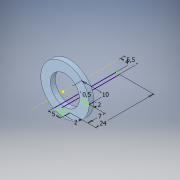
# Autodesk Inventor part: Zugentlastung
Saved by Autodesk Inventor 2018.2 (Build 222227000, 227)
## iProperties
Created: 2018-03-03
Part Number: Zugentlastung
Material: Generisch
Document SubType Name: Modeling
Designer: JochenAlt
Density: 1 g/cm^3
Appearance: Vorgabe
Author: JochenAlt
Autodesk Inventor part; units mm, degrees
ref_plane "YZ Plane" through (0, 0, 0) normal (1, 0, 0) x (0, 1, 0)
ref_plane "XZ Plane" through (0, 0, 0) normal (0, 1, 0) x (-1, 0, 0)
ref_plane "XY Plane" through (0, 0, 0) normal (0, 0, 1) x (1, 0, 0)
sketch "Skizze1" plane through (0, 0, 0) normal (0, 0, 1) x (1, 0, 0)
  line L0 (0, 23.0554) -> (0, -13.3446) construction
  line L1 (-2, 0) -> (12, 0) construction
  line L2 (4, 17.8554) -> (5.5, 17.8554)
  line L3 (5.5, 17.8554) -> (5.5, -6.1446)
  line L4 (4, 17.8554) -> (4, -8.1446)
  line L5 (4, -8.1446) -> (9, -8.1446)
  line L6 (9, -8.1446) -> (9, -6.1446)
  line L7 (9, -6.1446) -> (5.5, -6.1446)
  line L8 (6, 2.8554) -> (6, 0.8554)
  line L9 (6, 2.8554) -> (10, 2.8554)
  line L10 (10, 2.8554) -> (10, 0.8554)
  line L11 (10, 0.8554) -> (6, 0.8554)
  point P0 (0, 0)
  dimension "d9" = 4
  dimension "d10" = 5.5
  dimension "d11" = 5
  dimension "d12" = 2
  dimension "d13" = 24
  dimension "d14" = 0.5
  dimension "d15" = 2
  dimension "d16" = 10
  dimension "d21" = 7
  constraints: 20 end point, 4 perpendicular, 3 horizontal, 3 vertical
  measures "d9" distance between parallel lines of L4 L0
  measures "d10" distance between parallel lines of L0 L3
  measures "d11" distance between parallel lines of L6 L4
  measures "d12" distance between parallel lines of L5 L7
  measures "d13" distance between parallel lines of L7 L2
  measures "d14" distance between parallel lines of L3 L8
  measures "d15" distance between parallel lines of L11 L9
  measures "d16" distance between parallel lines of L10 L0
  measures "d21" distance between parallel lines of L11 L7
revolve "Umdrehung1" add sketch "Skizze1" angle 360 about axis through (0, 0, 0) along (0, -1, 0) contours L2 L3 L7 L6 L5 L4
revolve "Umdrehung2" add sketch "Skizze1" angle 360 about axis through (0, 0, 0) along (0, -1, 0) separate body contours L9 L10 L11 L8
